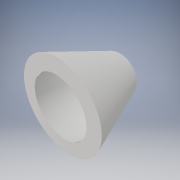
# Autodesk Inventor part: Socket
Saved by Autodesk Inventor 2017.2 (Build 212233000, 233)
## iProperties
Created: 2018-01-21
Part Number: Socket
Material: Generic
Document SubType Name: Modeling
Designer: Vatsal Varma
Density: 1 g/cm^3
Appearance: Default
Author: Vatsal Varma
Autodesk Inventor part; units mm, degrees
ref_plane "YZ Plane" through (0, 0, 0) normal (1, 0, 0) x (0, 1, 0)
ref_plane "XZ Plane" through (0, 0, 0) normal (0, 1, 0) x (-1, 0, 0)
sketch "Sketch1" plane through (0, 0, 0) normal (0, 0, 1) x (1, 0, 0)
  circle A0 centre (0, 0) radius 5
  dimension "d0" = 10
  constraints: 1 centre point, 1 coincident
  measures "d0" diameter of A0
ref_plane "Work Plane1" through (0, 0, -7.5) normal (0, 0, 1) x (1, 0, 0)
sketch "Sketch2" plane through (0, 0, -7.5) normal (0, 0, 1) x (1, 0, 0)
  circle A0 centre (0, 0) radius 2.5
  dimension "d2" = 5
  constraints: 1 centre point, 1 coincident
  measures "d2" diameter of A0
loft "Loft1" add profiles "Sketch1", "Sketch2"
sketch "Sketch3" plane through (0, 0, 0) normal (0, 1, 0) x (-1, 0, 0)
  arc A0 (0, 2.5) -> (0, -4.5) centre (0, -1) ccw
  line L0 (0, 5.5184) -> (0, -9.2276)
  line L1 (2.5, -7.5) -> (-2.5, -7.5) projected
  point P0 (0, 0)
  dimension "d7" = 7
  dimension "d9" = 1
  constraints: 3 point on line, 2 end point, 2 point on circle, 1 centre point, 1 perpendicular
  measures "d7" diameter of A0
  measures "d9" distance of A0.centre point (0, 0)
revolve "Revolution1" cut sketch "Sketch3" angle 360 about axis through (0, 0, 5.5184) along (0, 0, -1)
sketch "Sketch4" plane through (0, 0, -7.5) normal (0, 0, -1) x (-1, 0, 0)
  circle A0 centre (0, 0) radius 1
  dimension "d10" = 2
  constraints: 1 centre point, 1 coincident
  measures "d10" diameter of A0
extrude "Extrusion1" cut sketch "Sketch4" against normal blind 3
body "Solid1"
